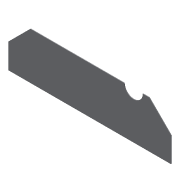
# Autodesk Inventor part: bladehalf
Saved by Autodesk Inventor 2015 (Build 190159000, 159)
## iProperties
Created: 2015-10-28
Part Number: bladehalf
Material: Generic
Document SubType Name: Modeling
Designer: jad211
Density: 1 g/cm^3
Appearance: Default
Author: jad211
Autodesk Inventor part; units mm, degrees
ref_plane "YZ Plane" through (0, 0, 0) normal (1, 0, 0) x (0, 1, 0)
ref_plane "XZ Plane" through (0, 0, 0) normal (0, 1, 0) x (-1, 0, 0)
ref_plane "XY Plane" through (0, 0, 0) normal (0, 0, 1) x (1, 0, 0)
sketch "Sketch1" plane through (0, 0, 0) normal (0, 1, 0) x (-1, 0, 0)
  line L0 (1.5, 0) -> (16.5, 0)
  line L1 (20, -3.5) -> (20, -7.5)
  line L2 (20, -7.5) -> (-6, -7.5)
  line L3 (-6, -7.5) -> (-6, -3.5)
  arc A0 (-1.5, 0) -> (1.5, 0) centre (0, 0) ccw
  line L4 (-2.5, 0) -> (-1.5, 0)
  line L5 (1.5, 0) -> (16.5, 0)
  line L6 (16.5, 0) -> (20, -3.5)
  line L7 (-2.5, 0) -> (-6, -3.5)
  point P0 (-9.6433, 0)
  dimension "d0" = 1.5
  dimension "d1" = 7.5
  dimension "d6" = 4
  dimension "d7" = 4
  dimension "d10" = 135
  dimension "d11" = 7.5
  dimension "d12" = 1
  dimension "d13" = 20
  constraints: 16 end point, 4 perpendicular, 3 collinear, 2 point on circle, 1 centre point, 1 coincident, 1 horizontal, 1 point on line
  measures "d0" radius of A0
  measures "d1" distance from line of L2 A0.centre
  measures "d6" distance of L1.start L1.end
  measures "d7" distance of L2.end L3.end
  measures "d10" angle of L1 L6
  measures "d11" distance between parallel lines of L2 L0
  measures "d12" distance of L4.start L4.end
  measures "d13" distance from line of point (0, 0) L1
extrude "Extrusion1" add sketch "Sketch1" along normal blind 0.1
equation "\"d7\" = d6"
equation "\"d11\" = d1"
body "Solid1"
